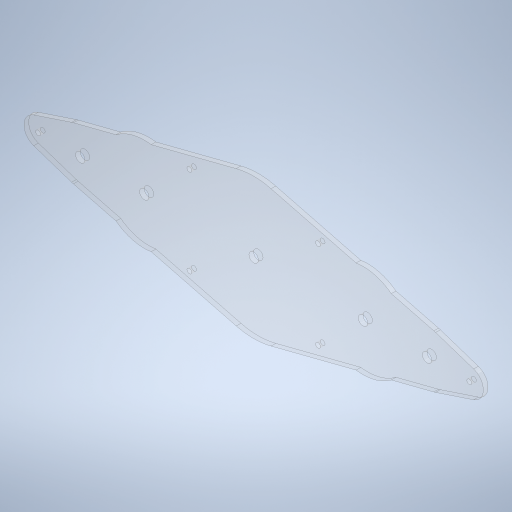
# Autodesk Inventor part: frame
Saved by Autodesk Inventor 2023 (Build 270158000, 158)
## iProperties
Created: 2023-05-29
Part Number: frame
Material: PMMA Plastic
Document SubType Name: Sheet Metal
Designer: Ronan
Density: 1.188 g/cm^3
Appearance: Polycarbonate - Clear
Sheet Metal Rule: Default_mm
Mass: 57.2053 g
Surface Area: 343.314 cm^2
Volume: 48.1526 cm^3
Author: Ronan
Autodesk Inventor part; units mm, degrees
ref_plane "YZ Plane" through (0, 0, 0) normal (1, 0, 0) x (0, 1, 0)
ref_plane "XZ Plane" through (0, 0, 0) normal (0, 1, 0) x (-1, 0, 0)
ref_plane "XY Plane" through (0, 0, 0) normal (0, 0, 1) x (1, 0, 0)
sketch "Sketch1" plane through (0, 0, 0) normal (0, 0, 1) x (1, 0, 0)
  circle A0 centre (0, 0) radius 45
  circle A1 centre (70, 0) radius 30
  circle A2 centre (111, 0) radius 17.5
  circle A3 centre (138, 0) radius 9
  circle A4 centre (-70, 0) radius 30
  circle A5 centre (-111, 0) radius 17.5
  circle A6 centre (-138, 0) radius 9
  line L0 (-11.1486, 43.5971) -> (-115.3356, 16.9544)
  line L1 (11.1486, 43.5971) -> (115.3356, 16.9544)
  line L2 (-116.5093, 16.6102) -> (-140.8333, 8.5424)
  line L3 (116.5093, 16.6102) -> (140.8333, 8.5424)
  line L4 (-11.1486, -43.5971) -> (-115.3356, -16.9544)
  line L5 (11.1486, -43.5971) -> (115.3356, -16.9544)
  line L6 (140.8333, -8.5424) -> (116.5093, -16.6102)
  line L7 (-140.8333, -8.5424) -> (-116.5093, -16.6102)
  circle A7 centre (-138, 0) radius 1.5
  circle A8 centre (-111, 0) radius 3
  circle A9 centre (-70, 0) radius 3
  circle A10 centre (0, 0) radius 3
  circle A11 centre (70, 0) radius 3
  circle A12 centre (111, 0) radius 3
  circle A13 centre (138, 0) radius 1.5
  line L8 (-123.0921, -97.5699) -> (-152.3126, 20.9991) construction
  line L9 (-152.3126, 20.9991) -> (130.841, 90.7804) construction
  line L10 (130.841, 90.7804) -> (160.0615, -27.7887) construction
  line L11 (160.0615, -27.7887) -> (-123.0921, -97.5699) construction
  circle A14 centre (-41.1855, -28.1747) radius 1.5
  circle A15 centre (-41.1855, 28.1747) radius 1.5
  circle A16 centre (41.1855, 28.1747) radius 1.5
  circle A17 centre (41.1855, -28.1747) radius 1.5
  line L12 (0, 45) -> (0, -45)
  line L13 (-37.7402, 24.5088) -> (37.7402, -24.5088)
  line L14 (-37.7402, -24.5088) -> (37.7402, 24.5088)
  line L15 (-45, 0) -> (45, 0)
  point P0 (-88.1111, 23.9163)
  point P1 (-88.1111, -23.9163)
  point P2 (-65.5931, -29.6746)
  point P3 (65.5931, -29.6746)
  point P4 (88.1111, -23.9163)
  point P5 (88.1111, 23.9163)
  point P6 (65.5931, 29.6746)
  point P7 (-65.5931, 29.6746)
  point P8 (0, 0)
  dimension "d0" = 90
  dimension "d1" = 60
  dimension "d2" = 70
  dimension "d3" = 35
  dimension "d4" = 41
  dimension "d5" = 18
  dimension "d6" = 27
  dimension "d7" = 0
  dimension "d8" = 0
  dimension "d9" = 0
  dimension "d10" = 60
  dimension "d11" = 35
  dimension "d12" = 41
  dimension "d13" = 18
  dimension "d16" = 70
  dimension "d17" = 0
  dimension "d18" = 0
  dimension "d19" = 0
  dimension "d20" = 27
  dimension "d23" = 6
  dimension "d24" = 6
  dimension "d25" = 6
  dimension "d26" = 3
  dimension "d27" = 6
  dimension "d28" = 6
  dimension "d29" = 3
  dimension "d109" = 0.5
  dimension "d121" = 7.5
  dimension "d133" = 3
  dimension "d138" = 8.8
  dimension "d139" = 3.4005
  dimension "d140" = 3
  dimension "d141" = 3
  dimension "d142" = 3
  dimension "d143" = 7.5
  dimension "d145" = 8.8
  dimension "d146" = 7.5
  dimension "d148" = 8.8
  dimension "d151" = 8.8
  dimension "d152" = 3.4005
  dimension "d153" = 3.4005
  dimension "d155" = 7.5
  dimension "d156" = 3.4005
  dimension "d157" = 57
  dimension "d159" = 57
  constraints: 24 end point, 17 centre point, 12 point on circle, 12 tangent, 8 coincident, 4 midpoint, 2 vertical, 1 horizontal, 21 other
  measures "d1" diameter of A1
  measures "d2" distance of point (0, 0) A1.centre
  measures "d3" diameter of A2
  measures "d4" distance of A1.centre A2.centre
  measures "d5" diameter of A3
  measures "d6" distance of A3.centre A2.centre
  measures "d7" vertical distance of point (0, 0) A3.centre
  measures "d8" vertical distance of point (0, 0) A2.centre
  measures "d9" vertical distance of point (0, 0) A1.centre
  measures "d10" diameter of A4
  measures "d11" diameter of A5
  measures "d12" distance of A4.centre A5.centre
  measures "d13" diameter of A6
  measures "d16" distance of A4.centre point (0, 0)
  measures "d17" vertical distance of point (0, 0) A4.centre
  measures "d18" vertical distance of point (0, 0) A5.centre
  measures "d19" vertical distance of point (0, 0) A6.centre
  measures "d20" distance of A5.centre A6.centre
  measures "d23" diameter of A10
  measures "d24" diameter of A11
  measures "d25" diameter of A12
  measures "d26" diameter of A13
  measures "d27" diameter of A9
  measures "d28" diameter of A8
  measures "d29" diameter of A7
  measures "d109" angle of L5 L11
  measures "d121" distance from line of L4 A14.centre
  measures "d133" diameter of A14
  measures "d140" diameter of A15
  measures "d141" diameter of A16
  measures "d142" diameter of A17
  measures "d143" distance from line of L0 A15.centre
  measures "d146" distance from line of L1 A16.centre
  measures "d155" distance from line of A17.centre L5
  measures "d157" angle of L14 L12
  measures "d159" angle of L12 L13
extrude "Extrusion1" add sketch "Sketch1" along normal blind 3 contours L14 A10 L12 A0 | A0 L1 A1 | A0 A1 L15 A10 L14 | A1 L1 A2 L5 A0 | A0 L15 A1 | L12 A10 L13 A0 | A1 L1 | A0 A1 L15 | A1 A0 L13 A10 L15 | A0 A4 L0 | L1 A2 A1 | A1 L5 A0 | L13 A0 L12 A10 | A10 L15 A4 A0 L13 | L12 A0 L14 A10 | L14 A0 A4 L15 A10 | L0 A4 | A4 A0 L4 A5 L0 | A2 A1 | A1 A2 | L5 A1 | A0 L4 A4 | L15 A0 A4 | A4 A0 L15 | A4 A5 L0 | A2 L5 A1 | L3 A3 L6 A2 | A5 A4 | A4 A5 | A3 | A4 L4 | A4 L4 A5 | A5 L7 A6 L2 | A6
equation "\"BendRadius\" = Thickness"
equation "\"BendReliefWidth\" = Thickness"
equation "\"BendReliefDepth\" = 0.5 * Thickness"
equation "\"CornerReliefSize\" = 4 * Thickness"
equation "\"MinimumRemnant\" = 2 * Thickness"
equation "\"TransitionRadius\" = BendRadius"
equation "\"JacobiRadiusSize\" = BendRadius"
equation "\"GapSize\" = Thickness"
equation "\"Thickness\" = 3"
body "Solid1"
